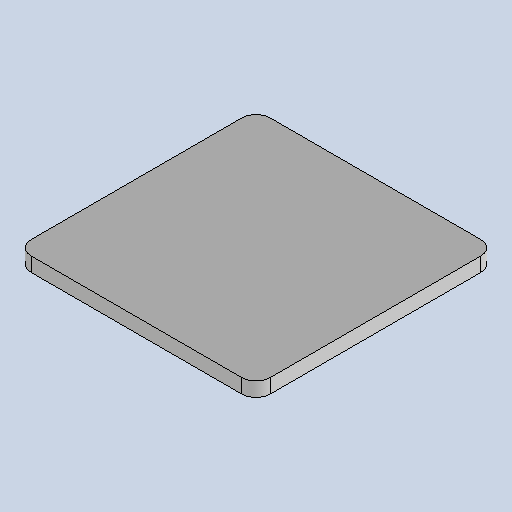
# Autodesk Inventor part: ANP 1426 FDS way cup
Saved by Autodesk Inventor 2025.3 (Build 293356030, 356C)
## iProperties
Created: 2025-06-24
Part Number: ANP 1426 FDS way cup
Material: Stainless Steel
Document SubType Name: Sheet Metal
Designer: user
Mass: 17.9011 g
Surface Area: 24.9877 cm^2
Volume: 2.23763 cm^3
Density: 8 g/cm^3
Flat Pattern Width: 3.35 cm
Flat Pattern Length: 3.35 cm
Flat Pattern Area: 11.2225 cm^2
Sheet Metal Rule: AISI304 2mm Die16
Sheet Metal Width: 33,500 mm
Sheet Metal Length: 33,500 mm
Sheet Metal Area: 1122,250 mm^2
Appearance: Default
Author: user
Autodesk Inventor part; units mm, degrees
ref_plane "YZ Plane" through (0, 0, 0) normal (1, 0, 0) x (0, 1, 0)
ref_plane "XZ Plane" through (0, 0, 0) normal (0, 1, 0) x (-1, 0, 0)
ref_plane "XY Plane" through (0, 0, 0) normal (0, 0, 1) x (1, 0, 0)
sketch "Sketch1" plane through (0, 0, 0) normal (0, 0, 1) x (1, 0, 0)
  line L0 (-16.75, -16.75) -> (16.75, -16.75)
  line L1 (16.75, -16.75) -> (16.75, 16.75)
  line L2 (16.75, 16.75) -> (-16.75, 16.75)
  line L3 (-16.75, 16.75) -> (-16.75, -16.75)
  line L4 (-16.75, -16.75) -> (16.75, 16.75) construction
  line L5 (16.75, -16.75) -> (-16.75, 16.75) construction
  point P0 (0, 0)
  dimension "d154" = 33.5
  dimension "d155" = 33.5
  measures "d154" distance of L1.end L2.end
  measures "d155" distance of L0.end L1.end
extrude "Plate5" add sketch "Sketch1" along normal blind 2
fillet "Corner Round1" radius 2 4 edges at (16.75, 16.75, 1) (-16.75, 16.75, 1) (-16.75, -16.75, 1) (16.75, -16.75, 1)
body "Solid3"
